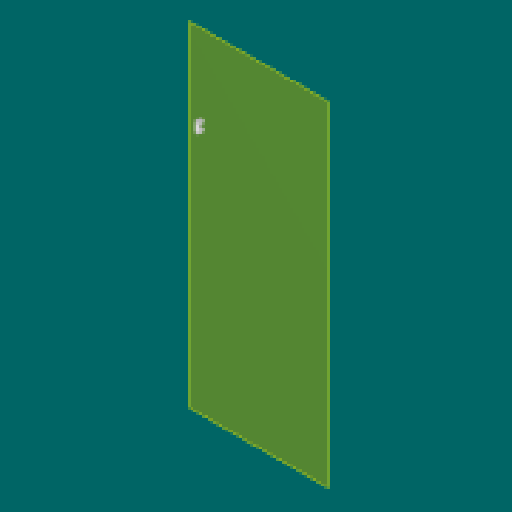
# Autodesk Inventor part: U_OS
Saved by Autodesk Inventor 2023 (Build 270158000, 158)
## iProperties
Created: 2023-01-28
Part Number: U_OS
Material: Generic
Document SubType Name: Modeling
Designer: HeavyDrewno
Density: 1 g/cm^3
Appearance: Default
Author: HeavyDrewno
Autodesk Inventor part; units mm, degrees
ref_plane "YZ Plane" through (0, 0, 0) normal (1, 0, 0) x (0, 1, 0)
ref_plane "XZ Plane" through (0, 0, 0) normal (0, 1, 0) x (-1, 0, 0)
ref_plane "XY Plane" through (0, 0, 0) normal (0, 0, 1) x (1, 0, 0)
ref_plane "Work Plane1" through (170, -244, 0) normal (0, 0, 1) x (1, 0, 0)
sketch "Sketch1" plane through (170, -244, 0) normal (0, 0, 1) x (1, 0, 0)
  line L0 (-170, 244) -> (-180, 244)
  line L1 (-180, 244) -> (-180, 276)
  line L2 (-180, 276) -> (-170, 276)
  line L3 (-170, 276) -> (-170, 244)
  dimension "d0" = 10
  dimension "d1" = 32
  constraints: 8 end point, 2 parallel, 1 horizontal, 1 perpendicular
  measures "d0" distance of L1.end L2.end
  measures "d1" distance of L0.end L1.end
extrude "Extrusion1" add sketch "Sketch1" along normal blind 16
sketch "Sketch2" plane through (-10, 0, 0) normal (-1, 0, 0) x (0, 0, 1)
  arc A0 (6, 10) -> (6, 22) centre (6, 16) ccw
  line L0 (0, 32) -> (16, 32) projected
  line L1 (0, 38.4) -> (0, -6.4) projected
  line L2 (6, 10) -> (0, 10)
  line L3 (0, 32) -> (0, 0) projected
  line L4 (6, 22) -> (0, 22)
  line L5 (0, 10) -> (0, 22)
  dimension "d4" = 12
  dimension "d5" = 16
  dimension "d6" = 6
  constraints: 6 end point, 2 point on circle, 2 point on line, 1 centre point, 1 collinear, 1 parallel, 1 perpendicular, 1 tangent
  measures "d4" diameter of A0
  measures "d5" distance from line of L0 A0.centre
  measures "d6" distance from line of L1 A0.centre
extrude "Extrusion2" cut sketch "Sketch2" against normal blind 16
sketch "Sketch3" plane through (170, -244, 16) normal (0, 0, 1) x (1, 0, 0)
  line L0 (-170, 244) -> (-170, 276) projected
  line L1 (-170, 276) -> (-180, 276) projected
  line L2 (-180, 244) -> (-170, 244) projected
  point P0 (-175, 249)
  point P1 (-175, 271)
  dimension "d9" = 5
  dimension "d10" = 5
  dimension "d11" = 5
  dimension "d12" = 5
  measures "d9" distance from line of L0 point (-175, 249)
  measures "d10" distance from line of L0 point (-175, 271)
  measures "d11" distance from line of L1 point (-175, 271)
  measures "d12" distance from line of L2 point (-175, 249)
hole "Hole1" at (-5, 5, 16) at (-5, 27, 16) direction (0, 0, -1) diameter 6.5 end through all
body "Solid1"
